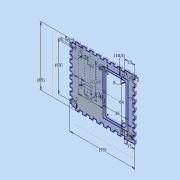
# Autodesk Inventor part: Bottom
Saved by Autodesk Inventor 2015 (Build 190159000, 159)
## iProperties
Created: 2015-01-28
Part Number: Bottom
Material: Wood (Birch)
Document SubType Name: Modeling
Designer: Openlab
Density: 0.55 g/cm^3
Appearance: Polycarbonate - Clear
Author: Openlab
Autodesk Inventor part; units mm, degrees
ref_plane "YZ Plane" through (0, 0, 0) normal (1, 0, 0) x (0, 1, 0)
ref_plane "XZ Plane" through (0, 0, 0) normal (0, 1, 0) x (-1, 0, 0)
ref_plane "XY Plane" through (0, 0, 0) normal (0, 0, 1) x (1, 0, 0)
sketch "Sketch1" plane through (0, 0, 0) normal (0, 1, 0) x (-1, 0, 0)
  line L0 (46, -10.5) -> (10, -10.5)
  line L1 (10, -10.5) -> (10, -74.5)
  line L2 (10, -74.5) -> (46, -74.5)
  line L3 (46, -74.5) -> (46, -10.5)
  line L4 (46, -10) -> (46, -55) construction
  line L5 (81, -55) -> (81, -10) construction
  line L6 (81, -10) -> (46, -10) construction
  line L7 (46, -55) -> (81, -55) construction
  line L8 (72.771, -10) -> (54.229, -10) construction
  line L9 (54.229, -10) -> (54.229, -53.18) construction
  line L10 (54.229, -53.18) -> (72.771, -53.18) construction
  line L11 (72.771, -53.18) -> (72.771, -10) construction
  line L12 (63.5, 3.8298) -> (63.5, -62.0489) construction
  line L13 (67.5, -15) -> (59.5, -15) construction
  line L14 (59.5, -15) -> (59.5, -10) construction
  line L15 (59.5, -10) -> (67.5, -10) construction
  line L16 (67.5, -10) -> (67.5, -15) construction
  circle A0 centre (77, -50) radius 3.5 construction
  circle A1 centre (50, -50) radius 3.5 construction
  circle A2 centre (77, -15) radius 3.5 construction
  circle A3 centre (50, -15) radius 3.5 construction
  line L17 (39, -13.5) -> (17, -13.5)
  line L18 (13, -17.5) -> (13, -67.5)
  line L19 (17, -71.5) -> (39, -71.5)
  line L20 (43, -67.5) -> (43, -17.5)
  line L21 (-0.7624, -103.1576) -> (89.2376, -103.1576) construction
  line L22 (117.4263, -3.5737) -> (117.4263, -83.5737) construction
  line L23 (0, 0) -> (0, -5)
  line L24 (0, -5) -> (3, -5)
  line L25 (3, -5) -> (3, -10)
  line L26 (3, -10) -> (0, -10)
  line L27 (0, -10) -> (0, -15)
  line L28 (0, -15) -> (3, -15)
  line L29 (3, -15) -> (3, -20)
  line L30 (3, -20) -> (0, -20)
  line L31 (0, -20) -> (0, -25)
  line L32 (0, -25) -> (3, -25)
  line L33 (3, -25) -> (3, -30)
  line L34 (3, -30) -> (0, -30)
  line L35 (0, -30) -> (0, -35)
  line L36 (0, -35) -> (3, -35)
  line L37 (3, -35) -> (3, -40)
  line L38 (3, -40) -> (0, -40)
  line L39 (0, -40) -> (0, -45)
  line L40 (0, -45) -> (3, -45)
  line L41 (3, -45) -> (3, -50)
  line L42 (3, -50) -> (0, -50)
  line L43 (0, -50) -> (0, -55)
  line L44 (0, -55) -> (3, -55)
  line L45 (3, -55) -> (3, -60)
  line L46 (3, -60) -> (0, -60)
  line L47 (0, -60) -> (0, -65)
  line L48 (0, -65) -> (3, -65)
  line L49 (3, -65) -> (3, -70)
  line L50 (3, -70) -> (0, -70)
  line L51 (0, -70) -> (0, -75)
  line L52 (0, -75) -> (3, -75)
  line L53 (3, -75) -> (3, -80)
  line L54 (0, 0) -> (15, 0)
  line L55 (15, 0) -> (15, -3)
  line L56 (15, -3) -> (20, -3)
  line L57 (20, -3) -> (20, 0)
  line L58 (20, 0) -> (25, 0)
  line L59 (25, 0) -> (25, -3)
  line L60 (25, -3) -> (30, -3)
  line L61 (30, -3) -> (30, 0)
  line L62 (30, 0) -> (35, 0)
  line L63 (35, 0) -> (35, -3)
  line L64 (35, -3) -> (40, -3)
  line L65 (40, -3) -> (40, 0)
  line L66 (40, 0) -> (45, 0)
  line L67 (45, 0) -> (45, -3)
  line L68 (45, -3) -> (50, -3)
  line L69 (50, -3) -> (50, 0)
  line L70 (50, 0) -> (55, 0)
  line L71 (55, 0) -> (55, -3)
  line L72 (55, -3) -> (60, -3)
  line L73 (60, -3) -> (60, 0)
  line L74 (60, 0) -> (65, 0)
  line L75 (65, 0) -> (65, -3)
  line L76 (65, -3) -> (70, -3)
  line L77 (70, -3) -> (70, 0)
  line L78 (70, 0) -> (75, 0)
  line L79 (75, 0) -> (75, -3)
  line L80 (75, -3) -> (80, -3)
  line L81 (80, -3) -> (80, 0)
  line L82 (80, 0) -> (85, 0)
  line L83 (93, -5) -> (93, -10)
  line L84 (93, -10) -> (90, -10)
  line L85 (90, -10) -> (90, -15)
  line L86 (90, -15) -> (93, -15)
  line L87 (93, -15) -> (93, -20)
  line L88 (93, -20) -> (90, -20)
  line L89 (90, -20) -> (90, -25)
  line L90 (90, -25) -> (93, -25)
  line L91 (93, -25) -> (93, -30)
  line L92 (93, -30) -> (90, -30)
  line L93 (90, -30) -> (90, -35)
  line L94 (90, -35) -> (93, -35)
  line L95 (93, -35) -> (93, -40)
  line L96 (93, -40) -> (90, -40)
  line L97 (90, -40) -> (90, -45)
  line L98 (90, -45) -> (93, -45)
  line L99 (93, -45) -> (93, -50)
  line L100 (93, -50) -> (90, -50)
  line L101 (90, -50) -> (90, -55)
  line L102 (90, -55) -> (93, -55)
  line L103 (93, -55) -> (93, -60)
  line L104 (93, -60) -> (90, -60)
  line L105 (90, -60) -> (90, -65)
  line L106 (3, -80) -> (0, -80)
  line L107 (0, -80) -> (0, -85)
  line L108 (0, -85) -> (15, -85)
  line L109 (15, -85) -> (15, -82)
  line L110 (15, -82) -> (20, -82)
  line L111 (20, -82) -> (20, -85)
  line L112 (20, -85) -> (25, -85)
  line L113 (25, -85) -> (25, -82)
  line L114 (25, -82) -> (30, -82)
  line L115 (30, -82) -> (30, -85)
  line L116 (30, -85) -> (35, -85)
  line L117 (35, -85) -> (35, -82)
  line L118 (35, -82) -> (40, -82)
  line L119 (40, -82) -> (40, -85)
  line L120 (40, -85) -> (45, -85)
  line L121 (45, -85) -> (45, -82)
  line L122 (45, -82) -> (50, -82)
  line L123 (50, -82) -> (50, -85)
  line L124 (50, -85) -> (55, -85)
  line L125 (55, -85) -> (55, -82)
  line L126 (55, -82) -> (60, -82)
  line L127 (60, -82) -> (60, -85)
  line L128 (60, -85) -> (65, -85)
  line L129 (65, -85) -> (65, -82)
  line L130 (65, -82) -> (70, -82)
  line L131 (70, -82) -> (70, -85)
  line L132 (70, -85) -> (75, -85)
  line L133 (75, -85) -> (75, -82)
  line L134 (75, -82) -> (80, -82)
  line L135 (80, -82) -> (80, -85)
  line L136 (80, -85) -> (85, -85)
  line L137 (14, -42.5) -> (78, -42.5) construction
  line L138 (46.5, -17.9001) -> (46.5, -65.4001) construction
  line L139 (90, -65) -> (93, -65)
  line L140 (93, -65) -> (93, -70)
  line L141 (93, -70) -> (90, -70)
  line L142 (90, -70) -> (90, -75)
  line L143 (90, -75) -> (93, -75)
  line L144 (93, -75) -> (93, -80)
  line L145 (85, 0) -> (85, -3)
  line L146 (85, -3) -> (90, -3)
  line L147 (85, -85) -> (85, -82)
  line L148 (85, -82) -> (90, -82)
  line L149 (93, -5) -> (90, -5)
  line L150 (90, -5) -> (90, -3)
  line L151 (93, -80) -> (90, -80)
  line L152 (90, -80) -> (90, -82)
  arc A4 (17, -13.5) -> (13, -17.5) centre (17, -17.5) ccw
  arc A5 (43, -17.5) -> (39, -13.5) centre (39, -17.5) ccw
  arc A6 (13, -67.5) -> (17, -71.5) centre (17, -67.5) ccw
  arc A7 (39, -71.5) -> (43, -67.5) centre (39, -67.5) ccw
  point P0 (85, -8)
  point P1 (85, -77)
  point P2 (8, -77)
  point P3 (8, -8)
  dimension "d72" = 10
  dimension "d2" = 36
  dimension "d3" = 64
  dimension "d22" = 35
  dimension "d24" = 5
  dimension "d25" = 4
  dimension "d26" = 5
  dimension "d27" = 4
  dimension "d28" = 18.542
  dimension "d29" = 43.18
  dimension "d30" = 8
  dimension "d31" = 5
  dimension "d34" = 7
  dimension "d35" = 7
  dimension "d36" = 7
  dimension "d37" = 7
  dimension "d41" = 3
  dimension "d42" = 3
  dimension "d43" = 3
  dimension "d44" = 3
  dimension "d87" = 15
  dimension "d126" = 5
  dimension "d127" = 3
  dimension "d128" = 5
  dimension "d129" = 3
  dimension "d130" = 3
  dimension "d131" = 5
  dimension "d132" = 15
  dimension "d134" = 7
  dimension "d144" = 5
  dimension "d146" = 45
  dimension "d147" = 5
  dimension "d148" = 3
  dimension "d149" = 5
  dimension "d150" = 5
  dimension "d151" = 5
  dimension "d152" = 5
  dimension "d153" = 5
  dimension "d154" = 5
  dimension "d155" = 5
  dimension "d156" = 5
  dimension "d164" = 69
  dimension "d165" = 8
  dimension "d166" = 10.5
  dimension "d167" = 85
  dimension "d168" = 93
  dimension "d170" = 10
  constraints: 306 end point, 105 perpendicular, 58 equal length, 49 collinear, 13 point on line, 11 horizontal, 10 parallel, 10 vertical, 8 centre point, 8 point on circle, 8 tangent, 5 horizontal alignment, 4 coincident, 3 vertical alignment, 6 other
  measures "d2" distance of L2.end L1.end
  measures "d3" distance of L1.end L0.end
  measures "d22" distance of L5.start L4.end
  measures "d24" distance from line of L6 point (77, -15)
  measures "d25" distance from line of L5 point (77, -50)
  measures "d26" distance from line of L7 point (77, -50)
  measures "d27" distance from line of L4 point (50, -15)
  measures "d28" distance of L9.end L10.end
  measures "d29" distance of L8.end L9.end
  measures "d30" distance of L13.start L13.end
  measures "d31" distance of L15.end L13.start
  measures "d34" diameter of A0
  measures "d35" diameter of A1
  measures "d36" diameter of A2
  measures "d37" diameter of A3
  measures "d41" distance between parallel lines of L0 L17
  measures "d42" distance between parallel lines of L3 L20
  measures "d43" distance between parallel lines of L1 L18
  measures "d44" distance between parallel lines of L2 L19
  measures "d87" distance of L23.start L54.end
  measures "d126" distance of L55.end L56.end
  measures "d127" distance of L54.end L55.end
  measures "d128" distance of L23.start L23.end
  measures "d129" distance of L23.end L24.end
  measures "d130" distance of L108.end L109.end
  measures "d131" distance of L109.end L110.end
  measures "d132" distance of L107.end L108.end
  measures "d134" distance between parallel lines of L37 L1
  measures "d144" distance of L83.start L83.end
  measures "d146" distance between parallel lines of L7 L6
  measures "d147" distance between parallel lines of L149 L82
  measures "d148" distance of L83.start L149.end
  measures "d149" distance from line of L146 point (85, -8)
  measures "d150" distance from line of L150 point (85, -8)
  measures "d151" distance from line of L148 point (85, -77)
  measures "d152" distance from line of L152 point (85, -77)
  measures "d153" distance from line of point (8, -77) L53
  measures "d154" distance from line of point (8, -77) L110
  measures "d155" distance from line of L25 point (8, -8)
  measures "d156" distance from line of L56 point (8, -8)
  measures "d164" distance of point (85, -77) point (85, -8)
  measures "d165" diameter of A4
  measures "d166" distance between parallel lines of L58 L0
  measures "d167" distance between parallel lines of L136 L82
  measures "d168" distance between parallel lines of L107 L144
  measures "d170" distance between parallel lines of L78 L6
extrude "Extrusion3" add sketch "Sketch1" along normal blind 3 contours L3 L2 L1 L0 | L54 L55 L56 L57 L58 L59 L60 L61 L62 L63 L64 L65 L66 L67 L68 L69 L70 L71 L72 L73 L74 L75 L76 L77 L78 L79 L80 L81 L82 L145 L146 L150 L149 L83 L84 L85 L86 L87 L88 L89 L90 L91 L92 L93 L94 L95 L96 L97 L98 L99 L100 L101 L102 L103 L104 L105 L139 L140 L141 L142 L143 L144 L151 L152 L148 L147 L136 L135 L134 L133 L132 L131 L130 L129 L128 L127 L126 L125 L124 L123 L122 L121 L120 L119 L118 L117 L116 L115 L114 L113 L112 L111 L110 L109 L108 L107 L106 L53 L52 L51 L50 L49 L48 L47 L46 L45 L44 L43 L42 L41 L40 L39 L38 L37 L36 L35 L34 L33 L32 L31 L30 L29 L28 L27 L26 L25 L24 L23
hole "Hole1" at (-77, 0, -50) at (-50, 0, -50) at (-50, 0, -15) at (-77, 0, -15) direction (0, 1, 0) diameter 3 end through all
hole "Hole2" at (-85, 0, -8) at (-85, 0, -77) at (-8, 0, -77) at (-8, 0, -8) direction (0, 1, 0) diameter 3 end through all
equation "\"x\" = 3"
body "Solid3"
